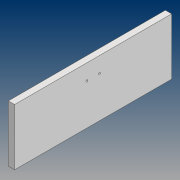
# Autodesk Inventor part: 09_Tam_canh_top_bottom
Saved by Autodesk Inventor 2021 (Build 250183000, 183)
## iProperties
Created: 2024-04-01
Part Number: 09_Tam_canh_top_bottom
Material: Generic
Document SubType Name: Modeling
Designer: Admin
Density: 1 g/cm^3
Appearance: Default
Author: Admin
Autodesk Inventor part; units mm, degrees
ref_plane "YZ Plane" through (0, 0, 0) normal (1, 0, 0) x (0, 1, 0)
ref_plane "XZ Plane" through (0, 0, 0) normal (0, 1, 0) x (-1, 0, 0)
ref_plane "XY Plane" through (0, 0, 0) normal (0, 0, 1) x (1, 0, 0)
sketch "Sketch1" plane through (0, 0, 0) normal (1, 0, 0) x (0, 1, 0)
  line L0 (-45, 125) -> (45, 125)
  line L1 (45, 125) -> (45, -125)
  line L2 (45, -125) -> (-45, -125)
  line L3 (-45, -125) -> (-45, 125)
  line L4 (-45, 125) -> (45, -125) construction
  line L5 (45, 125) -> (-45, -125) construction
  point P0 (0, 0)
  dimension "d0" = 250
  dimension "d1" = 90
  constraints: 12 end point, 2 midpoint, 2 parallel, 1 horizontal, 1 perpendicular
  measures "d0" distance of L0.end L1.end
  measures "d1" distance of L1.end L2.end
extrude "Extrusion1" add sketch "Sketch1" along normal blind 10
sketch "Sketch2" plane through (10, 0, 0) normal (1, 0, 0) x (0, 0, -1)
  line L0 (125, -45) -> (125, 45) projected
  line L1 (125, 45) -> (-125, 45) projected
  line L2 (-125, 45) -> (-125, -45) projected
  line L3 (-125, -45) -> (125, -45) projected
  line L4 (0, 45) -> (0, 20)
  line L5 (-10, 20) -> (10, 20)
  point P0 (0, 0)
  dimension "d4" = 20
  dimension "d5" = 25
  constraints: 4 end point, 2 midpoint, 1 horizontal, 1 symmetric about line, 1 vertical
  measures "d4" distance of L5.start L5.end
  measures "d5" distance of L4.start L4.end
hole "Hole1" at (10, 20, 10) at (10, 20, -10) direction (-1, 0, 0) diameter 3.2 end through all
body "Solid1"
